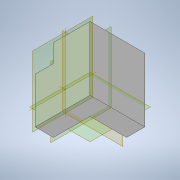
# Autodesk Inventor part: BT001_Winkel
Saved by Autodesk Inventor 2022 (Build 260153000, 153)
## iProperties
Created: 2022-01-02
Part Number: BT001_Winkel
Material: Generic
Document SubType Name: Modeling
Designer: Rayen
Density: 1 g/cm^3
Appearance: Default
Author: Rayen
Autodesk Inventor part; units mm, degrees
sketch "Sketch1" plane through (0, 0, 0) normal (1, 0, 0) x (0, 1, 0)
  line L0 (-188.502, 270.8493) -> (511.498, 270.8493)
  line L1 (511.498, 270.8493) -> (511.498, -129.1507)
  line L2 (511.498, -129.1507) -> (311.498, -129.1507)
  line L3 (311.498, -129.1507) -> (311.498, -329.1507)
  line L4 (311.498, -329.1507) -> (-188.502, -329.1507)
  line L5 (-188.502, -329.1507) -> (-188.502, 270.8493)
  point P0 (0, 0)
  dimension "d0" = 400
  dimension "d1" = 700
  dimension "d2" = 200
  dimension "d3" = 600
  constraints: 12 end point, 5 perpendicular, 1 horizontal
  measures "d0" distance of L0.end L1.end
  measures "d1" distance of L0.start L0.end
  measures "d2" distance of L1.end L2.end
  measures "d3" distance of L4.end L0.start
extrude "Extrusion1" add sketch "Sketch1" along normal blind 200
ref_plane "Work Plane1" through (200, 511.498, -129.1507) normal (1, 0, 0) x (0, 0, -1)
sketch "Sketch2" plane through (200, 511.498, -129.1507) normal (1, 0, 0) x (0, 0, -1)
  line L0 (-400, -700) -> (200, -700) projected
  line L1 (-400, -700) -> (-200, -700)
  line L2 (-200, -700) -> (-200, 0)
  line L3 (-400, 0) -> (-400, -700) projected
  line L4 (-200, 0) -> (-400, 0)
  line L5 (-400, 0) -> (-400, -700)
  point P0 (-129.1507, -511.498)
  dimension "d6" = 200
  dimension "d7" = 700
  constraints: 8 end point, 1 perpendicular, 1 point on line
  measures "d6" distance of L0.start L1.end
  measures "d7" distance of L1.end L2.end
extrude "Extrusion2" add sketch "Sketch2" along normal blind 400
body "Solid1"
